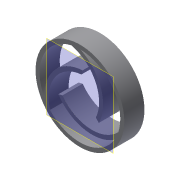
# Autodesk Inventor part: 10_P9_RMS_Fluofilter
Saved by Autodesk Inventor 2019 (Build 230136000, 136)
## iProperties
Created: 2019-08-22
Part Number: 10_P9_RMS_Fluofilter
Material: Generic
Document SubType Name: Modeling
Designer: diederichbenedict
Density: 1 g/cm^3
Appearance: Default
Author: diederichbenedict
Autodesk Inventor part; units mm, degrees
ref_plane "YZ Plane" through (0, 0, 0) normal (1, 0, 0) x (0, 1, 0)
ref_plane "Work Plane1" through (-20.25, 65.25, 45) normal (0, 0, -1) x (-1, 0, 0)
sketch "Sketch1" plane through (-20.25, 65.25, 45) normal (0, 0, -1) x (-1, 0, 0)
  circle A0 centre (0, 0) radius 15 construction
  circle A1 centre (0, 0) radius 15
  arc A2 (3.985843, 14.460742) -> (-9.363563, -1.43693) centre (8.57316, -2.944905) ccw
  arc A3 (-0.262145, 14.997709) -> (-11.417671, -3.55046) centre (8.57316, -2.944905) ccw
  circle A4 centre (0, 0) radius 17
  arc A5 (-3.177912, 14.659498) -> (-0.262145, 14.997709) centre (0, 0) ccw
  line L0 (-9.363563, -1.43693) -> (-11.417671, -3.55046)
  point P0 (-20.25, -65.25)
  dimension "d0" = 30
  dimension "d1" = 18
  dimension "d2" = 20
  dimension "d3" = 34
  constraints: 9 point on circle, 5 centre point, 3 coincident, 2 end point, 1 concentric
  measures "d0" diameter of A1
  measures "d1" radius of A2
  measures "d2" radius of A3
  measures "d3" diameter of A4
extrude "Extrusion1" add sketch "Sketch1" along normal blind 5 contours A2 L0 A3 A1 | A4 picked at (-9.618407, 0.814563)
pattern_circular "Circular Pattern1" count 3 over 360 about axis through (-20.25, 65.25, 45) along (0, 0, -1) of "Extrusion1"
sketch "Sketch2" plane through (-20.25, 65.25, 45) normal (0, 0, 1) x (1, 0, 0)
  circle A0 centre (0, 0) radius 17 projected
  circle A1 centre (0, 0) radius 15
  point P0 (20.25, -65.25)
  constraints: 1 centre point, 1 coincident
ref_plane "Work Plane2" through (-33.45, -70.55, 0) normal (0, 0, 1) x (1, 0, 0)
extrude "Extrusion2" add sketch "Sketch2" against normal up to surface (45 mm away)
sketch "Sketch3" plane through (-20.25, 65.25, 0) normal (0, 0, -1) x (-1, 0, 0)
  circle A0 centre (0, 0) radius 15 construction
  circle A1 centre (0, 0) radius 17 construction
  line L0 (15.2, -132.8) -> (15.2, 2.3)
  arc A2 (15.2, 2.3) -> (10.2, 7.3) centre (10.2, 2.3) ccw
  line L1 (10.2, 7.3) -> (-50.7, 7.3)
  circle A3 centre (0, 0) radius 17 construction
  arc A4 (13.11947, -7.271831) -> (3.985843, 14.460742) centre (0, 0) ccw construction
  arc A5 (15.2, -7.613147) -> (-15.35285, 7.3) centre (0, 0) ccw
  arc A6 (13.735534, 5.835534) -> (-13.103816, 7.3) centre (-0.038894, 0.06619) ccw
  point P0 (-20.25, -65.25)
  constraints: 6 point on circle, 3 point on line, 2 centre point, 8 other
ref_plane "Work Plane3" through (-33.45, -70.55, -7.1) normal (0, 0, -1) x (0, 1, 0)
extrude "Extrusion3" add sketch "Sketch3" along normal blind 9 contours L0 A2 A6 L1 A5
sketch "Sketch4" plane through (0, 0, 0) normal (1, 0, 0) x (0, 1, 0)
  line L0 (52.65, 10) -> (77.85, 10) construction
  line L1 (77.85, 15) -> (52.65, 15) construction
  line L2 (52.65, 10) -> (52.65, 15) construction
  line L3 (77.85, 10) -> (77.85, 15) construction
  line L4 (52.65, 10) -> (77.85, 10) construction
  line L5 (77.85, 10) -> (77.85, 15) construction
  line L6 (77.85, 15) -> (52.65, 15) construction
  line L7 (52.65, 15) -> (52.65, 10) construction
  line L8 (51.65, 16) -> (78.85, 16)
  line L9 (78.85, 16) -> (78.85, 9)
  line L10 (78.85, 9) -> (51.65, 9)
  line L11 (51.65, 9) -> (51.65, 16)
  point P0 (0, 0)
  dimension "d13" = 1
  constraints: 20 end point, 2 parallel, 2 perpendicular, 2 vertical, 1 horizontal, 3 other
  measures "d13" distance between parallel lines of L2 L11
extrude "Extrusion4" cut sketch "Sketch4" against normal through all
sketch "Sketch5" plane through (-26.577717, 51.65, 16) normal (0, 0, -1) x (-1, 0, 0)
  arc A0 (-19.431533, 20.9) -> (7.554064, 19.28297) centre (-6.327717, 13.6) ccw
  circle A1 centre (-6.327717, 13.6) radius 15
  circle A2 centre (-6.327717, 13.6) radius 10.935902
  point P0 (-26.577717, -51.65)
  constraints: 2 centre point, 2 coincident
extrude "Extrusion5" add sketch "Sketch5" against normal blind 3
fillet "Fillet1" radius 4 1 edges at (-35.25, 65.25, 19)
body "Solid1"
